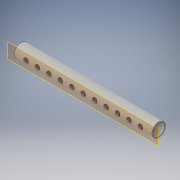
# Autodesk Inventor part: cArmPVC2inchSchedule40
Saved by Autodesk Inventor 2016 SP1 (Build 200210100, 210)
## iProperties
Created: 2016-01-12
Part Number: cArmPVC2inchSchedule40
Material: Generic
Document SubType Name: Modeling
Designer: steele
Density: 1 g/cm^3
Appearance: Default
Author: steele
Autodesk Inventor part; units mm, degrees
ref_plane "YZ Plane" through (0, 0, 0) normal (1, 0, 0) x (0, 1, 0)
ref_plane "XZ Plane" through (0, 0, 0) normal (0, 1, 0) x (-1, 0, 0)
sketch "Sketch3" plane through (0, 0, 0) normal (1, 0, 0) x (0, 1, 0)
  circle A0 centre (0, 0) radius 26.2509
  circle A1 centre (0, 0) radius 30.1625
  dimension "d10" = 60.325
  dimension "d11" = 52.5018
  constraints: 2 centre point, 2 coincident
  measures "d10" diameter of A1
  measures "d11" diameter of A0
extrude "Extrusion3" add sketch "Sketch3" along normal blind 609.6
ref_plane "Work Plane1" through (0, 0, 30.1625) normal (0, 0, 1) x (1, 0, 0)
sketch "Sketch4" plane through (0, 0, 30.1625) normal (0, 0, 1) x (1, 0, 0)
  circle A0 centre (50.8, 0) radius 10.668
  line L0 (0, 0) -> (611.1487, 0) construction
  circle A1 centre (101.6, 0) radius 10.668
  circle A2 centre (152.4, 0) radius 10.668
  circle A3 centre (203.2, 0) radius 10.668
  circle A4 centre (254, 0) radius 10.668
  circle A5 centre (304.8, 0) radius 10.668
  circle A6 centre (355.6, 0) radius 10.668
  circle A7 centre (406.4, 0) radius 10.668
  circle A8 centre (457.2, 0) radius 10.668
  circle A9 centre (508, 0) radius 10.668
  circle A10 centre (558.8, 0) radius 10.668
  line L1 (0, 30.1625) -> (0, -30.1625) projected
  dimension "d14" = 21.336
  dimension "d17" = 50.8
  dimension "d24" = 50.8
  constraints: 11 centre point, 2 end point, 2 horizontal, 20 other
  measures "d14" diameter of A0
  measures "d17" distance of A0.centre A1.centre
  measures "d24" distance from line of A0.centre L1
extrude "Extrusion4" cut sketch "Sketch4" against normal through all
equation "\"d10\" = cArmOutsideDiam"
equation "\"d11\" = cArmInsideDiam"
equation "\"d12\" = cArmLength"
equation "\"d14\" = cArmAxelHoleDaim"
equation "\"d17\" = cArmSpacing"
equation "\"d24\" = cArmSpacing"
equation "\"catapultArmWallThickness\" = 1.5875"
equation "\"catapultArmWidth\" = 50.8"
equation "\"catapultArmLength\" = 1219.2"
equation "\"cArmAxelHoleDaim\" = 21.336"
equation "\"catapultArmHoleDistanceFromEnd\" = 381"
equation "\"cArmInsideDiam\" = 52.5018"
equation "\"cArmOutsideDiam\" = 60.325"
equation "\"cArmLength\" = 609.6"
equation "\"cArmSpacing\" = 50.8"
body "Solid2"
